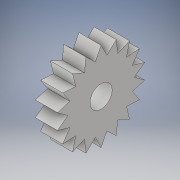
# Autodesk Inventor part: gear
Saved by Autodesk Inventor 2019 (Build 230136000, 136)
## iProperties
Created: 2018-11-15
Part Number: gear
Material: Generic
Document SubType Name: Modeling
Designer: Charlie
Density: 1 g/cm^3
Appearance: Default
Author: Charlie
Autodesk Inventor part; units mm, degrees
ref_plane "YZ Plane" through (0, 0, 0) normal (1, 0, 0) x (0, 1, 0)
ref_plane "XZ Plane" through (0, 0, 0) normal (0, 1, 0) x (-1, 0, 0)
ref_plane "XY Plane" through (0, 0, 0) normal (0, 0, 1) x (1, 0, 0)
sketch "Sketch2" plane through (0, 0, 0) normal (1, 0, 0) x (0, 1, 0)
  circle A0 centre (0, 0) radius 3.81
  line L0 (0, 0) -> (3.81, 0)
  line L1 (0, 0) -> (3.81, 0)
  line L2 (3.81, 0) -> (5.08, 0)
  line L3 (0, 0) -> (3.7521, -0.6616)
  line L4 (0, 0) -> (3.81, 0) construction
  line L5 (3.7521, -0.6616) -> (3.7521, 0.6616)
  line L6 (0, 0) -> (3.7521, 0.6616)
  line L7 (3.7521, 0.6616) -> (5.08, 0)
  line L8 (3.7521, -0.6616) -> (5.08, 0)
  line L9 (3.2996, 1.905) -> (4.7736, 1.7375)
  line L10 (3.5802, 1.3031) -> (4.7736, 1.7375)
  line L11 (3.7521, 0.6616) -> (4.7736, 1.7375)
  line L12 (3.7521, 0.6616) -> (3.2996, 1.905)
  line L13 (0, 0) -> (3.5802, 1.3031)
  line L14 (0, 0) -> (3.2996, 1.905)
  line L15 (0, 0) -> (3.7521, 0.6616)
  line L16 (2.449, 2.9186) -> (3.8915, 3.2654)
  line L17 (2.9186, 2.449) -> (3.8915, 3.2654)
  line L18 (3.2996, 1.905) -> (3.8915, 3.2654)
  line L19 (3.2996, 1.905) -> (2.449, 2.9186)
  line L20 (0, 0) -> (2.9186, 2.449)
  line L21 (0, 0) -> (2.449, 2.9186)
  line L22 (0, 0) -> (3.2996, 1.905)
  line L23 (1.3031, 3.5802) -> (2.54, 4.3994)
  line L24 (1.905, 3.2996) -> (2.54, 4.3994)
  line L25 (2.449, 2.9186) -> (2.54, 4.3994)
  line L26 (2.449, 2.9186) -> (1.3031, 3.5802)
  line L27 (0, 0) -> (1.905, 3.2996)
  line L28 (0, 0) -> (1.3031, 3.5802)
  line L29 (0, 0) -> (2.449, 2.9186)
  line L30 (0, 3.81) -> (0.8821, 5.0028)
  line L31 (0.6616, 3.7521) -> (0.8821, 5.0028)
  line L32 (1.3031, 3.5802) -> (0.8821, 5.0028)
  line L33 (1.3031, 3.5802) -> (0, 3.81)
  line L34 (0, 0) -> (0.6616, 3.7521)
  line L35 (0, 0) -> (0, 3.81)
  line L36 (0, 0) -> (1.3031, 3.5802)
  line L37 (-1.3031, 3.5802) -> (-0.8821, 5.0028)
  line L38 (-0.6616, 3.7521) -> (-0.8821, 5.0028)
  line L39 (0, 3.81) -> (-0.8821, 5.0028)
  line L40 (0, 3.81) -> (-1.3031, 3.5802)
  line L41 (0, 0) -> (-0.6616, 3.7521)
  line L42 (0, 0) -> (-1.3031, 3.5802)
  line L43 (0, 0) -> (0, 3.81)
  line L44 (-2.449, 2.9186) -> (-2.54, 4.3994)
  line L45 (-1.905, 3.2996) -> (-2.54, 4.3994)
  line L46 (-1.3031, 3.5802) -> (-2.54, 4.3994)
  line L47 (-1.3031, 3.5802) -> (-2.449, 2.9186)
  line L48 (0, 0) -> (-1.905, 3.2996)
  line L49 (0, 0) -> (-2.449, 2.9186)
  line L50 (0, 0) -> (-1.3031, 3.5802)
  line L51 (-3.2996, 1.905) -> (-3.8915, 3.2654)
  line L52 (-2.9186, 2.449) -> (-3.8915, 3.2654)
  line L53 (-2.449, 2.9186) -> (-3.8915, 3.2654)
  line L54 (-2.449, 2.9186) -> (-3.2996, 1.905)
  line L55 (0, 0) -> (-2.9186, 2.449)
  line L56 (0, 0) -> (-3.2996, 1.905)
  line L57 (0, 0) -> (-2.449, 2.9186)
  line L58 (-3.7521, 0.6616) -> (-4.7736, 1.7375)
  line L59 (-3.5802, 1.3031) -> (-4.7736, 1.7375)
  line L60 (-3.2996, 1.905) -> (-4.7736, 1.7375)
  line L61 (-3.2996, 1.905) -> (-3.7521, 0.6616)
  line L62 (0, 0) -> (-3.5802, 1.3031)
  line L63 (0, 0) -> (-3.7521, 0.6616)
  line L64 (0, 0) -> (-3.2996, 1.905)
  line L65 (-3.7521, -0.6616) -> (-5.08, 0)
  line L66 (-3.81, 0) -> (-5.08, 0)
  line L67 (-3.7521, 0.6616) -> (-5.08, 0)
  line L68 (-3.7521, 0.6616) -> (-3.7521, -0.6616)
  line L69 (0, 0) -> (-3.81, 0)
  line L70 (0, 0) -> (-3.7521, -0.6616)
  line L71 (0, 0) -> (-3.7521, 0.6616)
  line L72 (-3.2996, -1.905) -> (-4.7736, -1.7375)
  line L73 (-3.5802, -1.3031) -> (-4.7736, -1.7375)
  line L74 (-3.7521, -0.6616) -> (-4.7736, -1.7375)
  line L75 (-3.7521, -0.6616) -> (-3.2996, -1.905)
  line L76 (0, 0) -> (-3.5802, -1.3031)
  line L77 (0, 0) -> (-3.2996, -1.905)
  line L78 (0, 0) -> (-3.7521, -0.6616)
  line L79 (-2.449, -2.9186) -> (-3.8915, -3.2654)
  line L80 (-2.9186, -2.449) -> (-3.8915, -3.2654)
  line L81 (-3.2996, -1.905) -> (-3.8915, -3.2654)
  line L82 (-3.2996, -1.905) -> (-2.449, -2.9186)
  line L83 (0, 0) -> (-2.9186, -2.449)
  line L84 (0, 0) -> (-2.449, -2.9186)
  line L85 (0, 0) -> (-3.2996, -1.905)
  line L86 (-1.3031, -3.5802) -> (-2.54, -4.3994)
  line L87 (-1.905, -3.2996) -> (-2.54, -4.3994)
  line L88 (-2.449, -2.9186) -> (-2.54, -4.3994)
  line L89 (-2.449, -2.9186) -> (-1.3031, -3.5802)
  line L90 (0, 0) -> (-1.905, -3.2996)
  line L91 (0, 0) -> (-1.3031, -3.5802)
  line L92 (0, 0) -> (-2.449, -2.9186)
  line L93 (0, -3.81) -> (-0.8821, -5.0028)
  line L94 (-0.6616, -3.7521) -> (-0.8821, -5.0028)
  line L95 (-1.3031, -3.5802) -> (-0.8821, -5.0028)
  line L96 (-1.3031, -3.5802) -> (0, -3.81)
  line L97 (0, 0) -> (-0.6616, -3.7521)
  line L98 (0, 0) -> (0, -3.81)
  line L99 (0, 0) -> (-1.3031, -3.5802)
  line L100 (1.3031, -3.5802) -> (0.8821, -5.0028)
  line L101 (0.6616, -3.7521) -> (0.8821, -5.0028)
  line L102 (0, -3.81) -> (0.8821, -5.0028)
  line L103 (0, -3.81) -> (1.3031, -3.5802)
  line L104 (0, 0) -> (0.6616, -3.7521)
  line L105 (0, 0) -> (1.3031, -3.5802)
  line L106 (0, 0) -> (0, -3.81)
  line L107 (2.449, -2.9186) -> (2.54, -4.3994)
  line L108 (1.905, -3.2996) -> (2.54, -4.3994)
  line L109 (1.3031, -3.5802) -> (2.54, -4.3994)
  line L110 (1.3031, -3.5802) -> (2.449, -2.9186)
  line L111 (0, 0) -> (1.905, -3.2996)
  line L112 (0, 0) -> (2.449, -2.9186)
  line L113 (0, 0) -> (1.3031, -3.5802)
  line L114 (3.2996, -1.905) -> (3.8915, -3.2654)
  line L115 (2.9186, -2.449) -> (3.8915, -3.2654)
  line L116 (2.449, -2.9186) -> (3.8915, -3.2654)
  line L117 (2.449, -2.9186) -> (3.2996, -1.905)
  line L118 (0, 0) -> (2.9186, -2.449)
  line L119 (0, 0) -> (3.2996, -1.905)
  line L120 (0, 0) -> (2.449, -2.9186)
  line L121 (3.7521, -0.6616) -> (4.7736, -1.7375)
  line L122 (3.5802, -1.3031) -> (4.7736, -1.7375)
  line L123 (3.2996, -1.905) -> (4.7736, -1.7375)
  line L124 (3.2996, -1.905) -> (3.7521, -0.6616)
  line L125 (0, 0) -> (3.5802, -1.3031)
  line L126 (0, 0) -> (3.7521, -0.6616)
  line L127 (0, 0) -> (3.2996, -1.905)
  dimension "d3" = 7.62
  dimension "d12" = 1.27
  dimension "d13" = 10
  dimension "d16" = 360
  constraints: 256 end point, 3 horizontal, 3 point on circle, 1 centre point, 1 coincident, 1 collinear, 1 equal length, 1 vertical, 217 other
  measures "d3" diameter of A0
  measures "d12" distance of L0.end L2.end
  measures "d13" angle of L3 L4
extrude "Extrusion1" add sketch "Sketch2" along normal blind 2.54
sketch "Sketch3" plane through (2.54, 0, 0) normal (1, 0, 0) x (0, 0, -1)
  circle A0 centre (0, 0) radius 1.27
  dimension "d20" = 2.54
  constraints: 1 centre point, 1 coincident
  measures "d20" diameter of A0
extrude "Extrusion2" cut sketch "Sketch3" against normal blind 2.54
body "Solid1"
